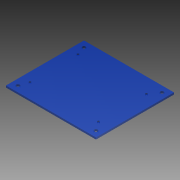
# Autodesk Inventor part: part_plate_rear
Saved by Autodesk Inventor 2014 (Build 180170000, 170)
## iProperties
Created: 2013-07-15
Part Number: part_plate_rear
Material: Polycarbonate, Clear
Document SubType Name: Modeling
Designer: Edward
Density: 1.2 g/cm^3
Appearance: Clear - Blue
Author: Edward
Autodesk Inventor part; units mm, degrees
ref_plane "YZ Plane" through (0, 0, 0) normal (1, 0, 0) x (0, 1, 0)
ref_plane "XZ Plane" through (0, 0, 0) normal (0, 1, 0) x (-1, 0, 0)
ref_plane "XY Plane" through (0, 0, 0) normal (0, 0, 1) x (1, 0, 0)
sketch "Sketch1" plane through (0, 0, 0) normal (0, 0, 1) x (1, 0, 0)
  line L0 (-75, 65) -> (75, 65)
  line L1 (75, 65) -> (75, -65)
  line L2 (75, -65) -> (-75, -65)
  line L3 (-75, -65) -> (-75, 65)
  point P0 (0, 0)
  dimension "d0" = 150
  dimension "d1" = 130
  dimension "d2" = 65
  dimension "d3" = 75
  constraints: 8 end point, 2 parallel, 1 horizontal, 1 perpendicular
  measures "d0" distance of L1.end L2.end
  measures "d1" distance of L0.end L1.end
  measures "d2" distance from line of point (0, 0) L0
  measures "d3" distance from line of L3 point (0, 0)
extrude "Extrusion1" add sketch "Sketch1" along normal blind 3
sketch "Sketch2" plane through (0, 0, 3) normal (0, 0, 1) x (1, 0, 0)
  circle A0 centre (-60, 40) radius 1.75
  line L0 (75, 65) -> (-75, 65) projected
  line L1 (-75, 65) -> (-75, -65) projected
  point P0 (0, 0)
  dimension "d6" = 3.5
  dimension "d15" = 25
  dimension "d16" = 15
  constraints: 1 centre point
  measures "d6" diameter of A0
  measures "d15" distance from line of L0 A0.centre
  measures "d16" distance from line of L1 A0.centre
extrude "Extrusion2" cut sketch "Sketch2" against normal through all
pattern_linear "Rectangular Pattern1" count 2 spacing 114 along (1, 0, 0) count 2 spacing 80 along (0, -1, 0) of "Extrusion2"
sketch "Sketch3" plane through (0, 0, 3) normal (0, 0, 1) x (1, 0, 0)
  line L0 (75, 65) -> (-75, 65) projected
  line L1 (-75, 65) -> (-75, -65) projected
  circle A0 centre (-65, 55) radius 2.75
  point P0 (0, 0)
  dimension "d17" = 5.5
  dimension "d18" = 10
  dimension "d19" = 10
  constraints: 1 centre point
  measures "d17" diameter of A0
  measures "d18" distance from line of L1 A0.centre
  measures "d19" distance from line of L0 A0.centre
extrude "Extrusion3" cut sketch "Sketch3" against normal through all
pattern_linear "Rectangular Pattern2" count 2 spacing 130 along (1, 0, 0) count 2 spacing 110 along (0, -1, 0) of "Extrusion3"
equation "\"d2\" = 0.5 * d1"
equation "\"d3\" = 0.5 * d0"
body "Solid1"
